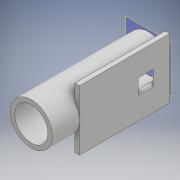
# Autodesk Inventor part: counter-adapter-USA-trap
Saved by Autodesk Inventor 2017 (Build 210142000, 142)
## iProperties
Created: 2018-06-27
Part Number: counter-adapter-USA-trap
Material: Generic
Document SubType Name: Modeling
Designer: 45027374
Density: 1 g/cm^3
Appearance: Default
Author: 45027374
Autodesk Inventor part; units mm, degrees
ref_plane "YZ Plane" through (0, 0, 0) normal (1, 0, 0) x (0, 1, 0)
ref_plane "XY Plane" through (0, 0, 0) normal (0, 0, 1) x (1, 0, 0)
sketch "Sketch1" plane through (0, 0, 0) normal (0, 1, 0) x (-1, 0, 0)
  line L0 (9.8, 0) -> (-9.8, 0) projected
  line L1 (0, -9.8) -> (0, 9.8) projected
  circle A0 centre (0, 0) radius 7
  circle A1 centre (0, 0) radius 5.5
  dimension "d0" = 14
  dimension "d1" = 11
  constraints: 2 centre point, 2 coincident
  measures "d0" diameter of A0
  measures "d1" diameter of A1
extrude "Extrusion1" add sketch "Sketch1" along normal blind 39 contours A0 L1 A1 L0 | L0 A1 L1 A0 | L1 A1 L0 A0 | A0 L0 A1 L1
ref_plane "Work Plane1" through (0, 39, 0) normal (0, 1, 0) x (-1, 0, 0)
sketch "Sketch4" plane through (0, 39, 0) normal (0, 1, 0) x (-1, 0, 0)
  circle A0 centre (0, 0) radius 7 projected
  circle A1 centre (0, 0) radius 5.5 projected
  line L0 (-7, -10) -> (-5.5, -10)
  line L1 (-5.5, -10) -> (-5.5, 10)
  line L2 (-5.5, 10) -> (-7, 10)
  line L3 (-7, 10) -> (-7, -10)
  line L4 (9.8, 0) -> (-9.8, 0) projected
  dimension "d10" = 20
  constraints: 8 end point, 2 parallel, 2 tangent, 1 horizontal, 1 perpendicular, 1 other
  measures "d10" distance of L2.end L0.start
extrude "Extrusion3" add sketch "Sketch4" against normal blind 30 contours L1 L4 A0 | A0 L3 L2 L1 | L1 L0 L3 A0 | A0 L4 L1
sketch "Sketch2" plane through (0, 0, 0) normal (1, 0, 0) x (0, 1, 0)
  line L0 (33.5, 2.5) -> (28.5, 2.5)
  line L1 (28.5, 2.5) -> (28.5, -2.5)
  line L2 (28.5, -2.5) -> (33.5, -2.5)
  line L3 (33.5, -2.5) -> (33.5, 2.5)
  line L4 (39, -7) -> (39, 7) projected
  line L5 (-7.8, 0) -> (46.8, 0) projected
  point P0 (0, 0)
  dimension "d4" = 5.5
  dimension "d5" = 5
  dimension "d6" = 5
  constraints: 8 end point, 2 parallel, 1 horizontal, 1 perpendicular, 1 other
  measures "d4" distance between parallel lines of L4 L3
  measures "d5" distance between parallel lines of L1 L3
  measures "d6" distance between parallel lines of L2 L0
extrude "Extrusion2" cut sketch "Sketch2" along normal through all
fillet "Fillet1" radius 3 6 edges at (4.899, 31, 2.5) (4.899, 31, -2.5) (5.3476, 28.5, -1.2856) (5.3476, 28.5, 1.2856) (5.3476, 33.5, -1.2856) (5.3476, 33.5, 1.2856)
body "Solid1"
